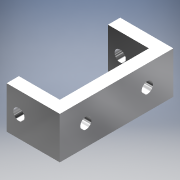
# Autodesk Inventor part: Bracket Sides
Saved by Autodesk Inventor 2019.4 (Build 234330000, 330)
## iProperties
Created: 2019-12-14
Part Number: Bracket Sides
Material: Aluminum 6061
Document SubType Name: Modeling
Designer: Mark
Mass: 17.6618 g
Surface Area: 32.9981 cm^2
Volume: 6.5414 cm^3
Density: 2.7 g/cm^3
Appearance: Aluminum - Flat
Author: Mark
Autodesk Inventor part; units mm, degrees
ref_plane "YZ Plane" through (0, 0, 0) normal (1, 0, 0) x (0, 1, 0)
ref_plane "XZ Plane" through (0, 0, 0) normal (0, 1, 0) x (-1, 0, 0)
ref_plane "XY Plane" through (0, 0, 0) normal (0, 0, 1) x (1, 0, 0)
sketch "Sketch1" plane through (0, 0, 0) normal (1, 0, 0) x (0, 1, 0)
  line L0 (-10.25, 27.75) -> (10.25, 27.75)
  line L1 (10.25, 27.75) -> (10.25, -27.75)
  line L2 (10.25, -27.75) -> (-10.25, -27.75)
  line L3 (-10.25, -27.75) -> (-10.25, 27.75)
  line L4 (-10.25, 27.75) -> (10.25, -27.75) construction
  line L5 (10.25, 27.75) -> (-10.25, -27.75) construction
  circle A0 centre (0, 15) radius 2.75
  circle A1 centre (0, -15) radius 2.75
  point P0 (0, 0)
  dimension "d0" = 20.5
  dimension "d1" = 55.5
  dimension "d2" = 5.5
  dimension "d3" = 5.5
  dimension "d4" = 30
  dimension "d5" = 10.25
  dimension "d6" = 12.75
  dimension "d7" = 10.25
  constraints: 12 end point, 2 centre point, 2 midpoint, 2 parallel, 1 horizontal, 1 perpendicular
  measures "d0" distance of L1.end L2.end
  measures "d1" distance of L0.end L1.end
  measures "d2" diameter of A0
  measures "d3" diameter of A1
  measures "d4" distance of A0.centre A1.centre
  measures "d5" distance from line of L3 A0.centre
  measures "d6" distance from line of L0 A0.centre
  measures "d7" distance from line of A1.centre L3
extrude "Extrusion1" add sketch "Sketch1" along normal blind 6
sketch "Sketch2" plane through (0, 0, 0) normal (-1, 0, 0) x (0, 0, 1)
  line L0 (27.75, -10.25) -> (-27.75, -10.25) projected
  line L1 (-27.75, -10.25) -> (-21.75, -10.25)
  line L2 (-21.75, -10.25) -> (-21.75, 10.25)
  line L3 (-21.75, 10.25) -> (-27.75, 10.25)
  line L4 (-27.75, 10.25) -> (-27.75, -10.25)
  line L5 (-27.75, 10.25) -> (27.75, 10.25) projected
  line L6 (27.75, 10.25) -> (21.75, 10.25)
  line L7 (21.75, 10.25) -> (21.75, -10.25)
  line L8 (21.75, -10.25) -> (27.75, -10.25)
  line L9 (27.75, -10.25) -> (27.75, 10.25)
  point P0 (0, 0)
  dimension "d10" = 6
  dimension "d11" = 20.5
  dimension "d12" = 6
  dimension "d13" = 20.5
  constraints: 16 end point, 4 parallel, 2 horizontal, 2 perpendicular
  measures "d10" distance of L3.end L2.end
  measures "d11" distance of L2.end L1.end
  measures "d12" distance of L8.end L7.end
  measures "d13" distance of L7.end L6.end
extrude "Extrusion2" add sketch "Sketch2" along normal blind 20 contours L0 L7 L5 L9 | L0 L4 L3 L2
sketch "Sketch3" plane through (6, -10.25, 27.75) normal (0, 0, 1) x (1, 0, 0)
  circle A0 centre (-15, 10.25) radius 2.75
  line L0 (0, 20.5) -> (0, 0) projected
  line L1 (-26, 0) -> (0, 0) projected
  point P0 (-6, 10.25)
  dimension "d16" = 5.5
  dimension "d17" = 15
  dimension "d18" = 10.25
  constraints: 1 centre point
  measures "d16" diameter of A0
  measures "d17" distance from line of L0 A0.centre
  measures "d18" distance from line of L1 A0.centre
extrude "Extrusion3" cut sketch "Sketch3" against normal blind 56.5125
body "Solid1"
